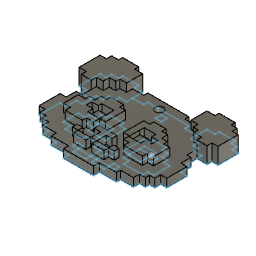
Homework-1 v2 (Autodesk Fusion 360 design; units mm, degrees)
Autodesk Fusion 360 part; units mm, degrees
sketch "panda" plane through (0, 0, 0) normal (0, 0, 1) x (1, 0, 0)
sketch "Sketch2" plane through (0, 0, 0) normal (0, 0, 1) x (1, 0, 0)
  line L0 (-22, 22) -> (-18, 22)
  line L1 (-18, 22) -> (-18, 21)
  line L2 (-18, 21) -> (-16, 21)
  line L3 (-16, 21) -> (-16, 18.5)
  line L4 (-16, 18.5) -> (-13.2496, 18.5)
  line L5 (-13.2496, 18.5) -> (-13.2496, 19.5)
  line L6 (-13.2496, 19.5) -> (-3, 19.5)
  line L7 (-3, 19.5) -> (-3, 18.5)
  line L8 (-3, 18.5) -> (0, 18.5)
  line L9 (0, 18.5) -> (0, 21)
  line L10 (0, 21) -> (2, 21)
  line L11 (2, 21) -> (2, 22)
  line L12 (2, 22) -> (6, 22)
  line L13 (6, 22) -> (6, 21)
  line L14 (6, 21) -> (7.5, 21)
  line L15 (7.5, 21) -> (7.5, 19.7623)
  line L16 (7.5, 19.7623) -> (9, 19.7623)
  line L17 (9, 19.7623) -> (9, 14.7196)
  line L18 (9, 14.7196) -> (7.5, 14.7196)
  line L19 (7.5, 14.7196) -> (7.5, 13.5)
  line L20 (7.5, 13.5) -> (5, 13.5)
  line L21 (5, 13.5) -> (5, 11)
  line L22 (5, 11) -> (6, 11)
  line L23 (6, 11) -> (6, 8.5)
  line L24 (6, 8.5) -> (7.5, 8.5)
  line L25 (7.5, 8.5) -> (7.5, 3.5)
  line L26 (7.5, 3.5) -> (6, 3.5)
  line L27 (6, 3.5) -> (6, 2)
  line L28 (6, 2) -> (4.7146, 2)
  line L29 (4.7146, 2) -> (4.7146, 1)
  line L30 (4.7146, 1) -> (3.2087, 1)
  line L31 (3.2087, 1) -> (3.2087, -0.5)
  line L32 (3.2087, -0.5) -> (0, -0.5)
  line L33 (0, -0.5) -> (0, -1.5)
  line L34 (0, -1.5) -> (-4.2468, -1.5)
  line L35 (-4.2468, -1.5) -> (-4.2468, -3)
  line L36 (-4.2468, -3) -> (-11.7023, -3)
  line L37 (-11.7023, -3) -> (-11.7023, -1.7302)
  line L38 (-11.7023, -1.7302) -> (-16, -1.7302)
  line L39 (-16, -1.7302) -> (-16, -0.5)
  line L40 (-16, -0.5) -> (-19.3059, -0.5)
  line L41 (-19.3059, -0.5) -> (-19.3059, 1)
  line L42 (-19.3059, 1) -> (-21, 1)
  line L43 (-21, 1) -> (-21, 2)
  line L44 (-21, 2) -> (-22.5, 2)
  line L45 (-22.5, 2) -> (-22.5, 3.2566)
  line L46 (-22.5, 3.2566) -> (-24, 3.2566)
  line L47 (-24, 3.2566) -> (-24, 8.5)
  line L48 (-24, 8.5) -> (-22.5, 8.5)
  line L49 (-22.5, 8.5) -> (-22.5, 11)
  line L50 (-22.5, 11) -> (-21, 11)
  line L51 (-21, 11) -> (-21, 13.2302)
  line L52 (-21, 13.2302) -> (-23.5, 13.2302)
  line L53 (-23.5, 13.2302) -> (-23.5, 14.5)
  line L54 (-23.5, 14.5) -> (-25.3048, 14.5)
  line L55 (-25.3048, 14.5) -> (-25.3048, 19.7229)
  line L56 (-25.3048, 19.7229) -> (-23.7249, 19.7229)
  line L57 (-23.7249, 19.7229) -> (-23.7249, 21)
  line L58 (-23.7249, 21) -> (-22, 21)
  line L59 (-22, 21) -> (-22, 22)
  line L60 (-21, 13.2302) -> (-21, 14.5)
  line L61 (-21, 14.5) -> (-19.3059, 14.5)
  line L62 (-19.3059, 14.5) -> (-19.3059, 16)
  line L63 (-19.3059, 16) -> (-17.7259, 16)
  line L64 (-17.7259, 16) -> (-17.7259, 17)
  line L65 (-17.7259, 17) -> (-16, 17)
  line L66 (-16, 17) -> (-16, 18.5)
  line L67 (-15, 12) -> (-15, 11)
  line L68 (-15, 11) -> (-16.2941, 11)
  line L69 (-16.2941, 11) -> (-16.2941, 9.5)
  line L70 (-16.2941, 9.5) -> (-17.7506, 9.5)
  line L71 (-17.7506, 9.5) -> (-17.7506, 8.5)
  line L72 (-17.7506, 8.5) -> (-19.5, 8.5)
  line L73 (-19.5, 8.5) -> (-19.5, 4.7872)
  line L74 (-19.5, 4.7872) -> (-17.7506, 4.7872)
  line L75 (-17.7506, 4.7872) -> (-17.7506, 3.5)
  line L76 (-17.7506, 3.5) -> (-13.5, 3.5)
  line L77 (-13.5, 3.5) -> (-13.5, 4.5)
  line L78 (-13.5, 4.5) -> (-11.7023, 4.5)
  line L79 (-11.7023, 4.5) -> (-11.7023, 6)
  line L80 (-11.7023, 6) -> (-10.2704, 6)
  line L81 (-10.2704, 6) -> (-10.2704, 11)
  line L82 (-10.2704, 11) -> (-11.7023, 11)
  line L83 (-11.7023, 11) -> (-11.7023, 12)
  line L84 (-11.7023, 12) -> (-15, 12)
  line L85 (-14.6453, 9.5265) -> (-14.6453, 8.6309)
  line L86 (-14.6453, 8.6309) -> (-11.7023, 8.6309)
  line L87 (-11.7023, 8.6309) -> (-11.7023, 9.5)
  line L88 (-11.7023, 9.5) -> (-14.6453, 9.5265)
  line L89 (-14.6453, 8.6309) -> (-14.6453, 6)
  line L90 (-14.6453, 6) -> (-11.7023, 6)
  line L91 (-11.7023, 6) -> (-11.7023, 8.6309)
  line L92 (-14.6453, 7.3155) -> (-16.2447, 7.3155)
  line L93 (-16.2447, 7.3155) -> (-16.2447, 8.6309)
  line L94 (-16.2447, 8.6309) -> (-14.6453, 8.6309)
  line L95 (-13.2504, 2.0158) -> (-13.2504, 0.8276)
  line L96 (-13.2504, 0.8276) -> (-11.8506, 0.8276)
  line L97 (-11.8506, 0.8276) -> (-11.8506, 2.0158)
  line L98 (-11.8506, 2.0158) -> (-13.2504, 2.0158)
  line L99 (-11.8506, 0.8276) -> (-11.8506, -0.3721)
  line L100 (-11.8506, -0.3721) -> (-8.7312, -0.3721)
  line L101 (-8.7312, -0.3721) -> (-8.7312, 0.8276)
  line L102 (-8.7312, 0.8276) -> (-11.8506, 0.8276)
  line L103 (-8.7312, 0.8276) -> (-8.7312, 3.2472)
  line L104 (-8.7312, 3.2472) -> (-10.2909, 3.2472)
  line L105 (-10.2909, 3.2472) -> (-10.2909, 4.5)
  line L106 (-10.2909, 4.5) -> (-5.8972, 4.5)
  line L107 (-5.8972, 4.5) -> (-5.8972, 3.2472)
  line L108 (-7.3114, 3.2472) -> (-5.8972, 3.2472)
  line L109 (-7.3114, 3.2472) -> (-7.3114, 0.8276)
  line L110 (-7.3114, 0.8276) -> (-8.7312, 0.8276)
  line L111 (-7.3114, 0.8276) -> (-7.3114, -0.3255)
  line L112 (-7.3114, -0.3255) -> (-4.292, -0.3255)
  line L113 (-4.292, -0.3255) -> (-4.292, 0.8276)
  line L114 (-4.292, 0.8276) -> (-7.3114, 0.8276)
  line L115 (-4.292, 0.8276) -> (-4.292, 2.0374)
  line L116 (-4.292, 2.0374) -> (-2.9107, 2.0374)
  line L117 (-2.9107, 2.0374) -> (-2.9107, 0.8276)
  line L118 (-2.9107, 0.8276) -> (-4.292, 0.8276)
  line L119 (-4.272, 12.0219) -> (-4.272, 11)
  line L120 (-4.272, 11) -> (-5.7517, 11)
  line L121 (-5.7517, 11) -> (-5.7517, 6)
  line L122 (-5.7517, 6) -> (-4.272, 6)
  line L123 (-4.272, 6) -> (-4.272, 4.5)
  line L124 (-4.272, 4.5) -> (-2.9374, 4.5)
  line L125 (-2.9374, 4.5) -> (-2.9374, 3.2272)
  line L126 (-2.9374, 3.2272) -> (1.727, 3.2272)
  line L127 (1.727, 3.2272) -> (1.727, 4.5)
  line L128 (1.727, 4.5) -> (3.2067, 4.5)
  line L129 (3.2067, 4.5) -> (3.2067, 8.5)
  line L130 (3.2067, 8.5) -> (1.727, 8.5)
  line L131 (1.727, 8.5) -> (1.727, 9.5)
  line L132 (1.727, 9.5) -> (0.2473, 9.5)
  line L133 (0.2473, 9.5) -> (0.2473, 11)
  line L134 (0.2473, 11) -> (-1.1925, 11)
  line L135 (-1.1925, 11) -> (-1.1925, 12.0219)
  line L136 (-1.1925, 12.0219) -> (-4.272, 12.0219)
  line L137 (-4.212, 9.6061) -> (-1.3325, 9.6061)
  line L138 (-1.3325, 9.6061) -> (-1.3325, 8.5)
  line L139 (-1.3325, 8.5) -> (-4.212, 8.5)
  line L140 (-4.212, 8.5) -> (-4.212, 9.6061)
  line L141 (-1.3325, 8.5) -> (-1.3325, 7)
  line L142 (-1.3325, 7) -> (0.2273, 7)
  line L143 (0.2273, 7) -> (0.2273, 8.5)
  line L144 (0.2273, 8.5) -> (-1.3325, 8.5)
  line L145 (-1.3325, 5.8068) -> (-1.3325, 8.5)
  line L146 (-4.212, 8.5) -> (-4.272, 6)
  line L147 (-1.3325, 5.8068) -> (-4.272, 5.8068)
  line L148 (0, 18.5) -> (0, 17)
  line L149 (0, 17) -> (1.767, 17)
  line L150 (1.767, 17) -> (1.767, 15.825)
  line L151 (1.767, 15.825) -> (3, 15.825)
  line L152 (3, 15.825) -> (3, 14.6852)
  line L153 (3, 14.6852) -> (5, 14.6852)
  line L154 (5, 14.6852) -> (5, 13.5)
  constraint horizontal L0
  constraint perpendicular L0 L1
  constraint perpendicular L1 L2
  constraint perpendicular L2 L3
  constraint perpendicular L3 L4
  constraint perpendicular L4 L5
  constraint perpendicular L5 L6
  constraint perpendicular L6 L7
  constraint perpendicular L7 L8
  constraint perpendicular L8 L9
  constraint perpendicular L9 L10
  constraint perpendicular L10 L11
  constraint perpendicular L11 L12
  constraint perpendicular L12 L13
  constraint perpendicular L13 L14
  constraint perpendicular L14 L15
  constraint perpendicular L15 L16
  constraint perpendicular L16 L17
  constraint perpendicular L17 L18
  constraint perpendicular L18 L19
  constraint perpendicular L19 L20
  constraint perpendicular L20 L21
  constraint perpendicular L21 L22
  constraint perpendicular L22 L23
  constraint perpendicular L23 L24
  constraint perpendicular L24 L25
  constraint perpendicular L25 L26
  constraint perpendicular L26 L27
  constraint perpendicular L27 L28
  constraint perpendicular L28 L29
  constraint perpendicular L29 L30
  constraint perpendicular L28 L31
  constraint perpendicular L31 L32
  constraint perpendicular L32 L33
  constraint perpendicular L33 L34
  constraint perpendicular L32 L35
  constraint perpendicular L33 L36
  constraint perpendicular L36 L37
  constraint perpendicular L37 L38
  constraint perpendicular L38 L39
  constraint perpendicular L39 L40
  constraint perpendicular L40 L41
  constraint perpendicular L41 L42
  constraint perpendicular L42 L43
  constraint perpendicular L43 L44
  constraint perpendicular L44 L45
  constraint perpendicular L45 L46
  constraint perpendicular L46 L47
  constraint perpendicular L47 L48
  constraint perpendicular L48 L49
  constraint perpendicular L49 L50
  constraint perpendicular L50 L51
  constraint perpendicular L51 L52
  constraint perpendicular L52 L53
  constraint perpendicular L51 L54
  constraint perpendicular L52 L55
  constraint perpendicular L55 L56
  constraint perpendicular L56 L57
  constraint perpendicular L57 L58
  constraint perpendicular L58 L59
  constraint perpendicular L52 L60
  constraint perpendicular L51 L61
  constraint perpendicular L52 L62
  constraint perpendicular L62 L63
  constraint perpendicular L63 L64
  constraint perpendicular L64 L65
  constraint perpendicular L65 L66
  constraint vertical L67
  constraint perpendicular L67 L68
  constraint perpendicular L68 L69
  constraint perpendicular L69 L70
  constraint perpendicular L70 L71
  constraint perpendicular L71 L72
  constraint perpendicular L70 L73
  constraint perpendicular L71 L74
  constraint perpendicular L70 L75
  constraint perpendicular L75 L76
  constraint perpendicular L76 L77
  constraint perpendicular L77 L78
  constraint perpendicular L76 L79
  constraint perpendicular L79 L80
  constraint perpendicular L76 L81
  constraint perpendicular L81 L82
  constraint perpendicular L82 L83
  constraint perpendicular L68 L85
  constraint perpendicular L85 L86
  constraint perpendicular L86 L87
  constraint perpendicular L86 L89
  constraint perpendicular L79 L90
  constraint perpendicular L86 L91
  constraint midpoint L89 L92.start
  constraint perpendicular L89 L92
  constraint perpendicular L92 L93
  constraint perpendicular L89 L94
  constraint perpendicular L76 L95
  constraint perpendicular L95 L96
  constraint perpendicular L76 L97
  constraint perpendicular L97 L98
  constraint perpendicular L96 L99
  constraint perpendicular L99 L100
  constraint perpendicular L100 L101
  constraint perpendicular L97 L102
  constraint perpendicular L102 L103
  constraint perpendicular L101 L104
  constraint perpendicular L102 L105
  constraint perpendicular L105 L106
  constraint horizontal L108
  constraint perpendicular L108 L109
  constraint perpendicular L107 L108
  constraint perpendicular L109 L110
  constraint perpendicular L110 L111
  constraint parallel L111 L113
  constraint perpendicular L109 L114
  constraint perpendicular L114 L115
  constraint perpendicular L115 L116
  constraint perpendicular L115 L118
  constraint perpendicular L111 L112
  constraint perpendicular L116 L117
  constraint vertical L119
  constraint perpendicular L119 L120
  constraint perpendicular L120 L121
  constraint perpendicular L121 L122
  constraint perpendicular L122 L123
  constraint perpendicular L123 L124
  constraint perpendicular L123 L126
  constraint perpendicular L126 L127
  constraint perpendicular L127 L128
  constraint perpendicular L128 L129
  constraint perpendicular L129 L130
  constraint perpendicular L130 L131
  constraint perpendicular L129 L132
  constraint perpendicular L130 L133
  constraint perpendicular L133 L134
  constraint perpendicular L134 L135
  constraint perpendicular L124 L125
  constraint perpendicular L135 L136
  constraint perpendicular L121 L137
  constraint perpendicular L137 L138
  constraint perpendicular L138 L139
  constraint perpendicular L139 L140
  constraint perpendicular L139 L141
  constraint perpendicular L141 L142
  constraint perpendicular L139 L143
  constraint perpendicular L143 L144
  constraint coincident L123 L147.end
  constraint perpendicular L123 L147
  constraint perpendicular L139 L145
  constraint perpendicular L8 L148
  constraint perpendicular L148 L149
  constraint perpendicular L149 L150
  constraint perpendicular L150 L151
  constraint perpendicular L151 L152
  constraint perpendicular L152 L153
  constraint perpendicular L20 L154
sketch "Sketch3" plane through (0, 0, 0) normal (0, 0, 1) x (1, 0, 0)
  line L0 (-8.859, 18.4208) -> (-8.859, 17)
  line L1 (-8.859, 17) -> (-7.3586, 17)
  line L2 (-7.3586, 17) -> (-7.3586, 18.4208)
  line L3 (-7.3586, 18.4208) -> (-8.859, 18.4208)
  constraint vertical L0
  constraint perpendicular L0 L1
  constraint perpendicular L1 L2
  constraint perpendicular L0 L3
extrude "Extrude1" add sketch "Sketch2" along normal blind 4 contours L0 L1 L2 L3 L52 L53 L54 L55 L56 L57 L58 L59 L60 L61 L62 L63 L64 L65 L66 makes body 1
extrude "Extrude2" add sketch "Sketch2" along normal blind 4 separate body contours L9 L10 L11 L12 L13 L14 L15 L16 L17 L18 L19 L20 L148 L149 L150 L151 L152 L153 L154 makes body 2
extrude "Extrude3" add sketch "Sketch2" along normal blind 4 separate body contours L103 L104 L105 L106 L107 L108 L109 L110 makes body 3
extrude "Extrude4" add sketch "Sketch2" along normal blind 4 separate body contours L111 L112 L113 L114 makes body 4
extrude "Extrude5" add sketch "Sketch2" along normal blind 4 separate body contours L115 L116 L117 L118 makes body 5
extrude "Extrude6" add sketch "Sketch2" along normal blind 4 separate body contours L99 L100 L101 L102 makes body 6
extrude "Extrude7" add sketch "Sketch2" along normal blind 4 separate body contours L95 L96 L97 L98 makes body 7
extrude "Extrude8" add sketch "Sketch2" along normal blind 4 separate body contours L119 L120 L121 L122 L123 L124 L125 L126 L127 L128 L129 L130 L131 L132 L133 L134 L135 L136 L137 L138 L140 L142 L143 L144 L145 L146 L147 makes body 8
extrude "Extrude9" add sketch "Sketch2" along normal blind 4 separate body contours L67 L68 L69 L70 L71 L72 L73 L74 L75 L76 L77 L78 L79 L80 L81 L82 L83 L84 makes body 9
extrude "Extrude10" add sketch "Sketch2" along normal blind 3 separate body contours L86 L89 L90 L91 makes body 10
extrude "Extrude11" add sketch "Sketch2" along normal blind 3 separate body contours L123 L139 L141 L145 L146 L147 makes body 11
extrude "Extrude12" add sketch "Sketch2" along normal blind 2 separate body contours L4 L5 L6 L7 L8 L21 L22 L23 L24 L25 L26 L27 L28 L29 L30 L31 L32 L33 L34 L35 L36 L37 L38 L39 L40 L41 L42 L43 L44 L45 L46 L47 L48 L49 L50 L51 L60 L61 L62 L63 L64 L65 L66 L148 L149 L150 L151 L152 L153 L154 makes body 12
extrude "Extrude13" add sketch "Sketch2" along normal blind 2 contours L137 L138 L139 L140 bodies 8 12 11
extrude "Extrude14" add sketch "Sketch2" along normal blind 2 separate body contours L141 L142 L143 L144 L145 makes body 13
extrude "Extrude15" add sketch "Sketch2" along normal blind 2 contours L85 L86 L87 L88 bodies 10 12 9
extrude "Extrude16" add sketch "Sketch2" along normal blind 2 separate body contours L89 L92 L93 L94 makes body 14
hole "Hole1" at (-8.233, 17.3798, 2) direction (0, 0, -1) diameter 2 depth 10 tip angle 118 bodies 12
combine "Combine1" operation add target body 1 tool bodies 2 8 13 10 14 3 5 12 6 7 4
